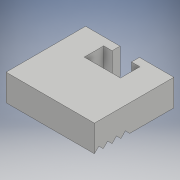
# Autodesk Inventor part: Clamp-part2(moving)-Base9x10mm.
Saved by Autodesk Inventor 2017 (Build 210142000, 142)
## iProperties
Created: 2021-08-04
Part Number: Clamp-part2(moving)-Base9x10mm.
Material: Generic
Document SubType Name: Modeling
Designer: Nikita
Density: 1 g/cm^3
Appearance: Default
Author: Nikita
Autodesk Inventor part; units mm, degrees
ref_plane "YZ Plane" through (0, 0, 0) normal (1, 0, 0) x (0, 1, 0)
ref_plane "XZ Plane" through (0, 0, 0) normal (0, 1, 0) x (-1, 0, 0)
ref_plane "XY Plane" through (0, 0, 0) normal (0, 0, 1) x (1, 0, 0)
sketch "Sketch1" plane through (0, 0, 0) normal (0, 0, 1) x (1, 0, 0)
  line L0 (0, 0) -> (10, 0)
  line L1 (10, 0) -> (10, 9)
  line L2 (10, 9) -> (0, 9)
  line L3 (0, 9) -> (0, 0)
  point P0 (5, 9)
  dimension "d0" = 10
  dimension "d1" = 9
  constraints: 8 end point, 2 parallel, 1 horizontal, 1 midpoint, 1 perpendicular
  measures "d0" distance of L2.end L1.end
  measures "d1" distance of L1.end L0.end
extrude "Extrusion1" add sketch "Sketch1" along normal blind 3
sketch "Sketch10" plane through (0, 0, 0) normal (-1, 0, 0) x (0, 0, 1)
  line L0 (0, 0) -> (3, 0) projected
  line L1 (3, 0) -> (2.5, 0)
  line L2 (2.5, 0) -> (2.5, 0.5)
  line L3 (2.5, 6) -> (3, 6)
  line L4 (3, 6) -> (3, 4)
  line L5 (3, 0) -> (3.7071, 0) construction
  line L6 (2.5, 4.25) -> (3, 4.25)
  line L7 (3, 1) -> (2.5, 1.5)
  line L8 (2.5, 1.5) -> (3, 2)
  line L9 (3, 2) -> (2.5, 2.5)
  line L10 (2.5, 2.5) -> (3, 3)
  line L11 (3, 3) -> (2.5, 3.5)
  line L12 (2.5, 3.5) -> (3, 4)
  line L13 (3, 4) -> (3, 4.25)
  line L14 (3, 1) -> (3, 0)
  line L15 (3, 2) -> (3, 1)
  line L16 (3, 4) -> (3, 3)
  line L17 (2.5, 2.5) -> (2.5, 3.5)
  line L18 (2.5, 1.5) -> (2.5, 2.5)
  line L19 (2.5, 0.5) -> (2.5, 1.5)
  line L20 (2.5, 3.5) -> (2.5, 6)
  line L21 (3, 3) -> (3, 2)
  line L22 (3, 1) -> (2.5, 0.5)
  line L23 (2.5, 0.5) -> (3, 0)
  point P0 (2.5, 3)
  dimension "d23" = 0.5
  dimension "d24" = 6
  constraints: 46 end point, 26 parallel, 11 perpendicular, 5 point on line, 2 horizontal
  measures "d23" distance of L3.end L3.start
  measures "d24" distance of L1.end L3.start
sketch "Sketch12" plane through (0, 0, 3) normal (0, 0, 1) x (1, 0, 0)
  line L0 (10, 9) -> (0, 9) projected
  line L1 (7.05, 5.9) -> (2.95, 5.9)
  line L2 (2.95, 5.9) -> (2.95, 8.1)
  line L3 (2.95, 8.1) -> (7.05, 8.1)
  line L4 (7.05, 8.1) -> (7.05, 5.9)
  line L5 (7.05, 5.9) -> (2.95, 8.1) construction
  line L6 (2.95, 5.9) -> (7.05, 8.1) construction
  line L7 (6.1, 7.2) -> (3.9, 7.2)
  line L8 (3.9, 7.2) -> (3.9, 9)
  line L9 (3.9, 9) -> (6.1, 9)
  line L10 (6.1, 9) -> (6.1, 7.2)
  line L11 (6.1, 7.2) -> (3.9, 9) construction
  line L12 (3.9, 7.2) -> (6.1, 9) construction
  line L13 (0, 9) -> (0, 0) projected
  point P0 (5, 7)
  point P1 (5, 8.1)
  dimension "d47" = 2
  dimension "d48" = 4.1
  dimension "d49" = 2.2
  dimension "d50" = 2.2
  dimension "d68" = 5
  constraints: 24 end point, 5 midpoint, 4 parallel, 2 horizontal, 2 perpendicular, 1 point on line
  measures "d47" distance from line of L0 point (5, 7)
  measures "d48" distance of L2.end L3.end
  measures "d49" distance of L1.end L2.end
  measures "d50" distance of L8.end L9.end
  measures "d68" distance from line of L13 point (5, 8.1)
extrude "Extrusion10" cut sketch "Sketch12" against normal up to next
extrude "Extrusion13" cut sketch "Sketch10" against normal up to next contours L23 L22 L14 | L7 L8 L15 | L9 L10 L21 | L11 L12 L16
body "Solid1"
